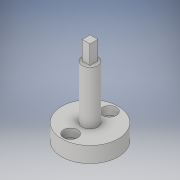
# Autodesk Inventor part: vex motor adaptor to tetrix
Saved by Autodesk Inventor 2019 (Build 230136000, 136)
## iProperties
Created: 2019-10-31
Part Number: vex motor adaptor to tetrix
Material: Generic
Document SubType Name: Modeling
Designer: User
Density: 1 g/cm^3
Appearance: Default
Author: User
Autodesk Inventor part; units mm, degrees
ref_plane "YZ Plane" through (0, 0, 0) normal (1, 0, 0) x (0, 1, 0)
ref_plane "XZ Plane" through (0, 0, 0) normal (0, 1, 0) x (-1, 0, 0)
ref_plane "XY Plane" through (0, 0, 0) normal (0, 0, 1) x (1, 0, 0)
sketch "Sketch1" plane through (0, 0, 0) normal (0, 1, 0) x (-1, 0, 0)
  circle A0 centre (0, 0) radius 11.43
  dimension "d0" = 22.86
  constraints: 1 centre point, 1 coincident
  measures "d0" diameter of A0
extrude "Extrusion1" add sketch "Sketch1" along normal blind 6.35
sketch "Sketch2" plane through (0, 6.35, 0) normal (0, 1, 0) x (1, 0, 0)
  point P0 (0, 0)
  point P1 (0, 7.8613)
  point P2 (0, -7.8613)
  dimension "d3" = 15.7226
  dimension "d4" = 7.8613
  measures "d3" distance of point (0, -7.861) point (0, 7.861)
  measures "d4" distance of point (0, 0) point (0, 7.861)
hole "Hole1" at (0, 6.35, -7.8613) at (0, 6.35, 7.8613) direction (0, -1, 0) diameter 3.4036 end through all counterbore diameter 5.715 counterbore depth 3.429
sketch "Sketch3" plane through (0, 6.35, 0) normal (0, 1, 0) x (1, 0, 0)
  circle A0 centre (0, 0) radius 3.175
  dimension "d12" = 6.35
  constraints: 1 centre point, 1 coincident
  measures "d12" diameter of A0
extrude "Extrusion2" add sketch "Sketch3" along normal blind 21.59
sketch "Sketch4" plane through (0, 27.94, 0) normal (0, 1, 0) x (1, 0, 0)
  line L0 (1.5875, -1.5875) -> (-1.5875, -1.5875)
  line L1 (-1.5875, -1.5875) -> (-1.5875, 1.5875)
  line L2 (-1.5875, 1.5875) -> (1.5875, 1.5875)
  line L3 (1.5875, 1.5875) -> (1.5875, -1.5875)
  point P0 (0, 0)
  dimension "d15" = 3.175
  dimension "d16" = 3.175
  dimension "d17" = 1.5875
  dimension "d18" = 1.5875
  constraints: 8 end point, 2 parallel, 1 horizontal, 1 perpendicular
  measures "d15" distance between parallel lines of L2 L0
  measures "d16" distance between parallel lines of L1 L3
  measures "d17" distance from line of L2 point (0, 0)
  measures "d18" distance from line of L3 point (0, 0)
extrude "Extrusion3" add sketch "Sketch4" along normal blind 7.62
equation "\"d4\" = 0.5 * d3"
equation "\"d17\" = 0.5 * d15"
equation "\"d18\" = 0.5 * d16"
body "Solid1"
